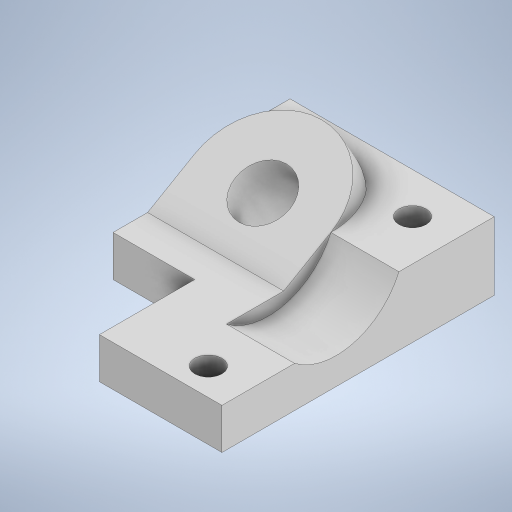
# Autodesk Inventor part: Pieza3-Tarea2
Saved by Autodesk Inventor 2024 (Build 280153000, 153)
## iProperties
Created: 2024-02-16
Part Number: Pieza3-Tarea2
Material: Genérico
Document SubType Name: Modeling
Designer: Diegolap
Density: 1 g/cm^3
Appearance: Valor por defecto
Mass: 118.902 g
Surface Area: 230.332 cm^2
Volume: 118.902 cm^3
Author: Diegolap
Autodesk Inventor part; units mm, degrees
ref_plane "YZ Plane" through (0, 0, 0) normal (1, 0, 0) x (0, 1, 0)
ref_plane "XZ Plane" through (0, 0, 0) normal (0, 1, 0) x (-1, 0, 0)
sketch "Boceto1" plane through (0, 0, 0) normal (0, 1, 0) x (-1, 0, 0)
  line L0 (-37.5, -50) -> (37.5, -50)
  line L1 (37.5, -50) -> (37.5, 50)
  line L2 (37.5, 50) -> (-37.5, 50)
  line L3 (-37.5, 50) -> (-37.5, -50)
  line L4 (-37.5, -50) -> (37.5, 50) construction
  line L5 (37.5, -50) -> (-37.5, 50) construction
  line L6 (37.5, 50) -> (7.5, 50)
  line L7 (7.5, 50) -> (7.5, 15)
  line L8 (7.5, 15) -> (37.5, 15)
  line L9 (37.5, 15) -> (37.5, 50)
  point P0 (0, 0)
  dimension "d0" = 100
  dimension "d1" = 75
  dimension "d2" = 30
  dimension "d3" = 35
  constraints: 20 end point, 4 parallel, 2 horizontal, 2 midpoint, 2 perpendicular
  measures "d0" distance of L0.end L1.end
  measures "d1" distance of L1.end L2.end
  measures "d2" distance of L7.end L8.end
  measures "d3" distance of L6.end L7.end
extrude "Extrusión1" add sketch "Boceto1" along normal blind 15 contours L3 L2 L7 L8 L1 L0
sketch "Boceto2" plane through (0, 15, 0) normal (0, 1, 0) x (1, 0, 0)
  line L0 (-37.5, 50) -> (-37.5, -15) projected
  line L1 (-37.5, 50) -> (37.5, 50)
  line L2 (37.5, 50) -> (37.5, 15)
  line L3 (37.5, 15) -> (-37.5, 15)
  line L4 (-37.5, 15) -> (-37.5, 50)
  point P0 (0, 0)
  dimension "d6" = 35
  dimension "d7" = 75
  constraints: 8 end point, 2 parallel, 1 horizontal, 1 perpendicular
  measures "d6" distance of L1.end L2.end
  measures "d7" distance of L2.end L3.end
extrude "Extrusión2" add sketch "Boceto2" along normal blind 10
ref_plane "Plano de trabajo1" through (-37.5, 25, -15) normal (0, -0.866, -0.5) x (1, 0, 0)
sketch "Boceto3" plane through (-37.5, 25, -15) normal (0, -0.866, -0.5) x (1, 0, 0)
  line L0 (75, 5) -> (75, 0) projected
  line L1 (75, 0) -> (50, 0)
  line L2 (0, 0) -> (75, 0) projected
  line L3 (0, 30.9808) -> (30, 30.9808) projected
  line L4 (0, 5) -> (0, 0) projected
  line L5 (0, 30.9808) -> (0, 0)
  arc A0 (0, 0) -> (50, 0) centre (25, 0) ccw
  line L6 (50, 0) -> (50, 30.9808)
  line L7 (50, 30.9808) -> (0, 30.9808)
  circle A1 centre (25, 0) radius 10
  point P0 (37.5, 25.4904)
  point P1 (0, 5)
  dimension "d11" = 25
  dimension "d12" = 20
  constraints: 8 end point, 2 centre point, 2 point on circle, 2 point on line, 2 tangent, 2 vertical, 1 coincident, 1 perpendicular
  measures "d11" distance of L1.end L0.end
  measures "d12" diameter of A1
extrude "Extrusión3" add sketch "Boceto3" along normal blind 10 contours A1 L2 L4 L5 L3 L7 L6 | L2 A0 A1
sketch "Boceto4" plane through (-37.5, 25, -15) normal (0, 0.866, 0.5) x (1, 0, 0)
  line L0 (15, 0) -> (35, 0) projected
  circle A0 centre (25, 0) radius 10
  point P0 (37.5, -25.4904)
  dimension "d15" = 20
  constraints: 1 centre point, 1 midpoint
  measures "d15" diameter of A0
extrude "Extrusión4" cut sketch "Boceto4" against normal blind 40
sketch "Boceto5" plane through (37.5, 0, 50) normal (1, 0, 0) x (0, 0, -1)
  line L0 (35, 15) -> (0, 15) projected
  line L1 (0, 15) -> (0, 10)
  line L2 (0, 0) -> (0, 15) projected
  line L3 (0, 10) -> (69.9738, 10)
  line L4 (100, 0) -> (100, 25) projected
  line L5 (65, 25) -> (47.6795, 15) projected
  line L6 (65, 15) -> (65, 25) projected
  arc A0 (62.0755, 49.9347) -> (65, 25) centre (41.9437, 34.9347) ccw
  circle A1 centre (41.9437, 34.9347) radius 25.1056
  line L7 (0, 15) -> (65, 15) projected
  circle A2 centre (41.9437, 34.9347) radius 30.4793
  line L8 (65, 25) -> (70.7584, 25)
  line L9 (65, 25) -> (100, 25) projected
  point P0 (50, 0)
  point P1 (57.2047, 15)
  point P2 (62.0755, 49.9347)
  point P3 (39.0192, 10)
  point P4 (44.8682, 10)
  dimension "d18" = 5
  constraints: 7 end point, 4 point on circle, 3 centre point, 2 coincident, 2 point on line, 1 concentric, 1 horizontal
  measures "d18" distance of L1.end L0.end
extrude "Extrusión5" add sketch "Boceto5" against normal blind 25 contours L7 A0 L3 L0 | L0 A0 A1 L5 L7 | L5 A0 L7 | L6 L7 A0
sketch "Boceto6" plane through (37.5, 0, 50) normal (1, 0, 0) x (0, 0, -1)
  arc A0 (65, 25) -> (26.6827, 15) centre (41.9437, 34.9347) ccw projected
  circle A1 centre (41.9437, 34.9347) radius 25.1056
  point P0 (50, 0)
  point P1 (26.6827, 15)
  constraints: 1 centre point, 1 coincident
extrude "Extrusión6" cut sketch "Boceto6" against normal blind 25
sketch "Boceto7" plane through (-37.5, 25, -15) normal (0, -0.866, -0.5) x (1, 0, 0)
  point P0 (37.5, 25.4904)
sketch "Boceto8" plane through (0, 25, 0) normal (0, 1, 0) x (1, 0, 0)
  circle A0 centre (22.5, 35) radius 5
  line L0 (37.5, 50) -> (-37.5, 50) projected
  line L1 (37.5, 15) -> (37.5, 50) projected
  circle A1 centre (22.5, -40) radius 5
  line L2 (-7.5, -50) -> (37.5, -50) projected
  line L3 (37.5, -50) -> (37.5, -23.3173) projected
  point P0 (0, 0)
  dimension "d23" = 15
  dimension "d24" = 15
  dimension "d25" = 10
  dimension "d26" = 10
  dimension "d27" = 15
  dimension "d28" = 10
  constraints: 2 centre point
  measures "d23" distance from line of L0 A0.centre
  measures "d24" distance from line of L1 A0.centre
  measures "d25" diameter of A0
  measures "d26" distance from line of L2 A1.centre
  measures "d27" distance from line of L3 A1.centre
  measures "d28" diameter of A1
extrude "Extrusión7" cut sketch "Boceto8" against normal blind 25
